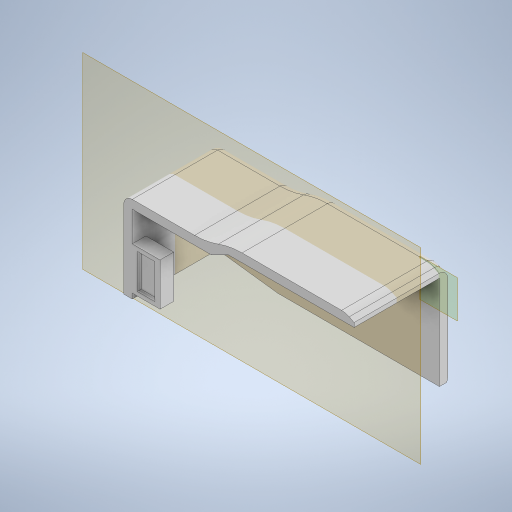
# Autodesk Inventor part: gondola
Saved by Autodesk Inventor 2023 (Build 270158000, 158)
## iProperties
Created: 2023-09-16
Part Number: gondola
Material: Generic
Document SubType Name: Modeling
Designer: alexa
Density: 1 g/cm^3
Appearance: Default
Author: alexa
Autodesk Inventor part; units mm, degrees
ref_plane "YZ Plane" through (0, 0, 0) normal (1, 0, 0) x (0, 1, 0)
ref_plane "XZ Plane" through (0, 0, 0) normal (0, 1, 0) x (-1, 0, 0)
ref_plane "XY Plane" through (0, 0, 0) normal (0, 0, 1) x (1, 0, 0)
sketch "Sketch1" plane through (0, 0, 0) normal (0, 1, 0) x (-1, 0, 0)
  line L0 (-70, 30) -> (70, 30)
  line L1 (70, 30) -> (70, -30)
  line L2 (70, -30) -> (-70, -30)
  line L3 (-70, -30) -> (-70, 30)
  line L4 (-70, 30) -> (70, -30) construction
  line L5 (70, 30) -> (-70, -30) construction
  point P0 (0, 0)
  dimension "d0" = 140
  dimension "d1" = 60
  constraints: 12 end point, 2 midpoint, 2 parallel, 1 horizontal, 1 perpendicular
  measures "d0" distance of L1.end L2.end
  measures "d1" distance between parallel lines of L0 L2
extrude "Extrusion1" add sketch "Sketch1" along normal blind 60
sketch "Sketch2" plane through (0, 60, 0) normal (0, 1, 0) x (1, 0, 0)
  point P0 (0, 0)
sketch "Sketch3" plane through (0, 60, 0) normal (0, 1, 0) x (1, 0, 0)
  line L0 (70, 30) -> (-70, 30) projected
  line L1 (-70, -30) -> (70, -30) projected
  line L2 (70, 30) -> (-20, 30)
  line L3 (-20, 30) -> (-20, -30)
  line L4 (-20, -30) -> (70, -30)
  line L5 (70, -30) -> (70, 30)
  point P0 (0, 0)
  point P1 (70, -30)
  point P2 (-20, 30)
  dimension "d4" = 90
  constraints: 8 end point, 2 parallel, 1 horizontal, 1 perpendicular, 1 point on line
  measures "d4" distance of L4.end L3.end
extrude "Extrusion2" add sketch "Sketch3" along normal blind 5
chamfer "Chamfer2" distance 5 distance2 40 1 edges at (-70, 0, 0) measured on face at (-70, 20, -10)
sketch "Sketch8" plane through (70, 0, 30) normal (1, 0, 0) x (0, 0, -1)
  circle A0 centre (30, 32.5) radius 13.25
  line L0 (0, 0) -> (60, 0) projected
  line L1 (60, 0) -> (60, 65) projected
  line L2 (0, 65) -> (60, 65) projected
  point P0 (30, 0)
  point P1 (60, 32.5)
  dimension "d26" = 26.5
  dimension "d27" = 32.5
  dimension "d28" = 30
  dimension "d88" = 32.5
  constraints: 1 centre point, 1 midpoint
  measures "d26" diameter of A0
  measures "d27" distance from line of L0 A0.centre
  measures "d28" distance of point (60, 32.5) A0.centre
  measures "d88" distance from line of L2 A0.centre
extrude "Extrusion6" cut sketch "Sketch8" against normal blind 10
sketch "Sketch9" plane through (70, 0, -30) normal (0, 0, -1) x (-1, 0, 0)
  line L0 (5, 60) -> (5, 5)
  line L1 (5, 5) -> (99.688711, 5)
  line L2 (99.688711, 5) -> (135, 9.413911)
  line L3 (135, 9.413911) -> (135, 55)
  line L4 (135, 55) -> (88.81966, 55)
  line L5 (88.81966, 55) -> (78.81966, 60)
  line L6 (78.81966, 60) -> (5, 60)
  line L7 (0, 65) -> (90, 65)
  line L8 (50, 80) -> (90, 60)
  line L9 (90, 60) -> (140, 60)
  line L10 (140, 5) -> (140, 60)
  line L11 (140, 5) -> (100, 0)
  line L12 (0, 0) -> (100, 0)
  line L13 (0, 0) -> (0, 65)
  point P0 (70, 0)
  dimension "d35" = 5
  dimension "d36" = 5
  dimension "d37" = 5
  dimension "d38" = 5
  dimension "d39" = 5
  dimension "d40" = 5
  dimension "d41" = 5
  constraints: 14 end point, 7 parallel, 2 perpendicular, 1 horizontal, 1 vertical, 1 other
  measures "d36" distance between parallel lines of L13 L0
  measures "d37" distance between parallel lines of L10 L3
  measures "d38" distance between parallel lines of L9 L4
  measures "d39" distance between parallel lines of L8 L5
  measures "d40" distance between parallel lines of L11 L2
  measures "d41" distance between parallel lines of L12 L1
extrude "Extrusion7" cut sketch "Sketch9" against normal blind 55 contours L6 L5 L4 L3 L2 L1 L0
ref_plane "Work Plane1" through (70, 0, 0) normal (0, 0, 1) x (1, 0, 0)
fillet "Fillet6" radius 5 1 edges at (-70, 60, 0)
fillet "Fillet9" radius 5 1 edges at (-70, 5, 0)
fillet "Fillet21" radius 40 1 edges at (-20, 65, 0)
fillet "Fillet22" radius 40 1 edges at (-20, 60, 0)
chamfer "Chamfer3" distance 10 distance2 5 1 edges at (70, 65, 0) measured on face at (46.455, 65, 10)
fillet "Fillet23" radius 5 1 edges at (70, 60, 0)
fillet "Fillet24" radius 10 1 edges at (60, 65, 0)
chamfer "Chamfer4" distance 5 distance2 10 1 edges at (70, 0, 0) measured on face at (70, 6.4489, -0.5324)
fillet "Fillet25" radius 10 1 edges at (60, 0, 0)
fillet "Fillet26" radius 5 1 edges at (70, 5, 0)
fillet "Fillet27" radius 5 15 edges at (59.9368, 64.7325, 30) (64.6738, 62.6631, 30) (69.2533, 59.5385, 30) (70, 32.5, 30) (69.2533, 5.4615, 30) (64.6738, 2.3369, 30) (59.9368, 0.2675, 30) (13.8197, 0, 30) (-7.7062, 64.37, 30) (-21.4028, 60.63, 30) (-46.737, 60, 30) (-70, 32.207, 30) (-68.7484, 6.1049, 30) (-47.8101, 2.2263, 30) (28.5021, 65, 30)
ref_plane "Work Plane7" through (65, 55, -24.5) normal (0, 0, -1) x (-1, 0, 0)
sketch "Sketch24" plane through (65, 55, -24.5) normal (0, 0, -1) x (-1, 0, 0)
  line L0 (0, 0) -> (5, 0) projected
  line L1 (5, 5) -> (5, 0) projected
  line L2 (5, 0) -> (5, 5) projected
  line L3 (0, 0) -> (0, 5) projected
  line L4 (5, 5) -> (0, 0)
  line L5 (5, -45) -> (5, -50) projected
  line L6 (0, -45) -> (5, -45) projected
  line L7 (0, -50) -> (0, -45) projected
  line L8 (0, -45) -> (5, -50)
  point P0 (65, -55)
  constraints: 4 end point
extrude "Extrusion21" cut sketch "Sketch24" against normal blind 5
sketch "Sketch27" plane through (65, 5, -30) normal (-1, 0, 0) x (0, 0, 1)
  line L0 (8.5, 30) -> (13.5, 30)
  line L1 (13.5, 30) -> (13.5, 25)
  line L2 (13.5, 25) -> (8.5, 25)
  line L3 (8.5, 25) -> (8.5, 30)
  line L4 (8.5, 30) -> (13.5, 25) construction
  line L5 (13.5, 30) -> (8.5, 25) construction
  circle A0 centre (30, 27.5) radius 13.25 projected
  line L6 (30, 73) -> (30, -18) projected
  line L7 (51.5, 30) -> (46.5, 30)
  line L8 (46.5, 30) -> (46.5, 25)
  line L9 (46.5, 25) -> (51.5, 25)
  line L10 (51.5, 25) -> (51.5, 30)
  point P0 (30, -5)
  point P1 (11, 27.5)
  dimension "d137" = 0
  dimension "d138" = 19
  dimension "d139" = 5
  dimension "d140" = 5
  constraints: 20 end point, 4 symmetric about line, 2 midpoint, 2 parallel, 1 horizontal, 1 perpendicular
  measures "d137" vertical distance of A0.centre point (11, 27.5)
  measures "d138" distance of A0.centre point (11, 27.5)
  measures "d139" distance of L2.end L0.start
  measures "d140" distance of L0.start L0.end
extrude "Extrusion24" add sketch "Sketch27" along normal blind 10 contours L0 L1 L2 L3 | L10 L9 L8 L7
sketch "Sketch28" plane through (65, 30, 16.5) normal (0, 0, -1) x (-1, 0, 0)
  line L0 (0, 5) -> (10, 5) projected
  line L1 (0, 0) -> (10, 0) projected
  line L2 (10, 5) -> (5, 5)
  line L3 (5, 5) -> (5, 0)
  line L4 (5, 0) -> (10, 0)
  line L5 (10, 0) -> (10, 5)
  point P0 (65, -30)
  point P1 (5, 5)
  dimension "d143" = 5
  constraints: 8 end point, 2 parallel, 1 horizontal, 1 midpoint, 1 perpendicular
  measures "d143" distance between parallel lines of L5 L3
extrude "Extrusion25" add sketch "Sketch28" along normal up to surface (33 mm away)
sketch "Sketch29" plane through (55, 5, -30) normal (-1, 0, 0) x (0, 0, 1)
  line L0 (30, 73) -> (30, -18) projected
  circle A0 centre (25.5, 27.5) radius 1.5
  line L1 (51.5, 30) -> (8.5, 30) projected
  line L2 (8.5, 25) -> (51.5, 25) projected
  circle A1 centre (34.5, 27.5) radius 1.5
  point P0 (30, -5)
  dimension "d146" = 4.5
  dimension "d147" = 3
  dimension "d148" = 2.5
  dimension "d149" = 2.5
  constraints: 2 centre point, 1 symmetric about line, 1 other
  measures "d146" distance from line of A0.centre L0
  measures "d147" diameter of A0
  measures "d148" distance from line of L1 A0.centre
  measures "d149" distance from line of L2 A0.centre
extrude "Extrusion26" cut sketch "Sketch29" against normal up to surface (5 mm away)
sketch "Sketch30" plane through (55, 5, -30) normal (-1, 0, 0) x (0, 0, 1)
  line L0 (30, 73) -> (30, -18) projected
  circle A0 centre (30, 27.5) radius 3.5
  line L1 (51.5, 30) -> (8.5, 30) projected
  point P0 (30, -5)
  dimension "d152" = 2.5
  dimension "d153" = 7
  constraints: 1 centre point, 1 midpoint
  measures "d152" distance from line of L1 A0.centre
  measures "d153" diameter of A0
extrude "Extrusion27" cut sketch "Sketch30" against normal up to surface (5 mm away)
sketch "Sketch32" plane through (0, 0, 0) normal (0, -1, 0) x (1, 0, 0)
  circle A0 centre (20, 0) radius 14.25
  line L0 (65, -30) -> (65, 25) projected
  point P0 (0, 0)
  point P1 (65, -21.5)
  dimension "d158" = 28.5
  dimension "d159" = 45
  constraints: 1 centre point
  measures "d158" diameter of A0
  measures "d159" distance from line of A0.centre L0
extrude "Extrusion29" cut sketch "Sketch32" against normal blind 5
ref_plane "Work Plane4" through (0, 32.5, 0) normal (0, -1, 0) x (1, 0, 0)
sketch "Sketch34" plane through (-29.688711, 5, -30) normal (0, 1, 0) x (1, 0, 0)
  line L0 (15.188711, -15.5) -> (8.188711, -15.5)
  line L1 (8.188711, -15.5) -> (8.188711, -8.5)
  line L2 (8.188711, -8.5) -> (15.188711, -8.5)
  line L3 (15.188711, -8.5) -> (15.188711, -15.5)
  line L4 (15.188711, -15.5) -> (8.188711, -8.5) construction
  line L5 (8.188711, -15.5) -> (15.188711, -8.5) construction
  line L6 (127.688711, -30) -> (-68.311289, -30)
  circle A0 centre (49.688711, -30) radius 14.25
  line L7 (15.188711, -44.5) -> (8.188711, -44.5)
  line L8 (8.188711, -44.5) -> (8.188711, -51.5)
  line L9 (8.188711, -51.5) -> (15.188711, -51.5)
  line L10 (15.188711, -51.5) -> (15.188711, -44.5)
  point P0 (29.688711, -30)
  point P1 (11.688711, -12)
  dimension "d163" = 7
  dimension "d164" = 7
  dimension "d166" = 18
  dimension "d167" = 38
  constraints: 20 end point, 4 symmetric about line, 2 midpoint, 2 parallel, 1 horizontal, 1 perpendicular
  measures "d163" distance between parallel lines of L2 L0
  measures "d164" distance between parallel lines of L1 L3
  measures "d166" distance from line of L6 point (11.689, -12)
  measures "d167" horizontal distance of A0.centre point (11.689, -12)
extrude "Extrusion30" add sketch "Sketch34" along normal blind 12 contours L0 L1 L2 L3 | L10 L9 L8 L7
sketch "Sketch35" plane through (-29.688711, 17, -30) normal (0, 1, 0) x (1, 0, 0)
  circle A0 centre (11.688711, -48) radius 2
  line L0 (8.188711, -44.5) -> (8.188711, -51.5)
  line L1 (15.188711, -44.5) -> (8.188711, -44.5)
  line L2 (15.188711, -51.5) -> (15.188711, -44.5)
  line L3 (127.688711, -30) -> (-68.311289, -30)
  circle A1 centre (11.688711, -12) radius 2
  point P0 (29.688711, -30)
  dimension "d170" = 4
  dimension "d171" = 3.5
  dimension "d172" = 3.5
  dimension "d173" = 3.5
  constraints: 2 centre point, 1 symmetric about line, 1 other
  measures "d170" diameter of A0
  measures "d171" distance from line of A0.centre L0
  measures "d172" distance from line of L1 A0.centre
  measures "d173" distance from line of L2 A0.centre
extrude "Extrusion31" cut sketch "Sketch35" against normal blind 5
sketch "Sketch37" plane through (-29.688711, 5, -30) normal (0, 1, 0) x (1, 0, 0)
  line L0 (8.188711, -51.5) -> (8.188711, -44.5)
  line L1 (0, -55) -> (94.688711, -55)
  line L2 (8.188711, -51.5) -> (15.188711, -51.5)
  line L3 (15.188711, -51.5) -> (15.188711, -55)
  line L4 (15.188711, -55) -> (8.188711, -55)
  line L5 (8.188711, -55) -> (8.188711, -51.5)
  line L6 (15.188711, -44.5) -> (15.188711, -51.5)
  point P0 (29.688711, -30)
  point P1 (8.188711, -55)
  dimension "d178" = 0
  constraints: 8 end point, 2 parallel, 1 collinear, 1 horizontal, 1 perpendicular, 1 point on line
  measures "d178" distance between parallel lines of L6 L3
extrude "Extrusion32" add sketch "Sketch37" along normal blind 12
sketch "Sketch38" plane through (65, 30, 21.5) normal (0, 0, 1) x (1, 0, 0)
  line L0 (0, 5) -> (0, 0) projected
  line L1 (0, 5) -> (-10, 5) projected
  line L2 (-10, 0) -> (-10, 5) projected
  line L3 (0, 0) -> (-10, 0) projected
  point P0 (-65, -30)
extrude "Extrusion33" add sketch "Sketch38" along normal up to surface (3.5 mm away)
ref_plane "Work Plane6" through (-70, 9.413911, -22.5) normal (0, 0, -1) x (-1, 0, 0)
ref_plane "Work Plane5" through (-70, 9.413911, -15) normal (0, 0, -1) x (-1, 0, 0)
sketch "Sketch42" plane through (55, 5, -30) normal (-1, 0, 0) x (0, 0, 1)
  line L0 (22.5, 34) -> (37.5, 34)
  line L1 (37.5, 34) -> (37.5, 21)
  line L2 (37.5, 21) -> (22.5, 21)
  line L3 (22.5, 21) -> (22.5, 34)
  arc A0 (32.44949, 25) -> (33.361111, 26.523818) centre (30, 27.5) ccw
  line L4 (22.5, 34) -> (37.5, 21) construction
  line L5 (37.5, 34) -> (22.5, 21) construction
  point P0 (30, -5)
  dimension "d193" = 15
  dimension "d194" = 13
  constraints: 12 end point, 2 midpoint, 2 parallel, 1 horizontal, 1 perpendicular
  measures "d193" distance of L0.start L0.end
  measures "d194" distance of L0.end L1.end
extrude "Extrusion36" add sketch "Sketch42" against normal blind 5
sketch "Sketch43" plane through (55, 5, -30) normal (-1, 0, 0) x (0, 0, 1)
  line L0 (24, 32.5) -> (36, 32.5)
  line L1 (36, 32.5) -> (36, 22.5)
  line L2 (36, 22.5) -> (24, 22.5)
  line L3 (24, 22.5) -> (24, 32.5)
  circle A0 centre (30, 27.5) radius 2.15 projected
  line L4 (24, 32.5) -> (36, 22.5) construction
  line L5 (36, 32.5) -> (24, 22.5) construction
  point P0 (30, -5)
  dimension "d197" = 12
  dimension "d199" = 10
  constraints: 12 end point, 2 midpoint, 2 parallel, 1 horizontal, 1 perpendicular
  measures "d197" distance of L0.start L0.end
  measures "d199" distance of L0.end L1.end
extrude "Extrusion37" cut sketch "Sketch43" against normal blind 2.5
sketch "Sketch44" plane through (55, 5, -30) normal (-1, 0, 0) x (0, 0, 1)
  line L0 (22.5, 25) -> (22.5, 21) projected
  line L1 (8.5, 25) -> (22.5, 25) projected
  line L2 (22.5, 21) -> (18.5, 25)
  point P0 (30, -5)
  dimension "d202" = 45
  dimension "d203" = 45
  constraints: 2 end point, 1 point on line
  measures "d202" angle of L1 L2
  measures "d203" angle of L0 L2
extrude "Extrusion38" add sketch "Sketch44" against normal blind 5
mirror "Mirror1" about plane through (70, 0, 0) normal (0, 0, 1) of "Extrusion38"
sketch "Sketch45" plane through (55, 5, -30) normal (-1, 0, 0) x (0, 0, 1)
  line L0 (37.5, 34) -> (22.5, 34) projected
  line L1 (22.5, 34) -> (18.5, 30)
  line L2 (8.5, 30) -> (22.5, 30) projected
  line L3 (22.5, 34) -> (22.5, 30) projected
  point P0 (30, -5)
  dimension "d206" = 45
  dimension "d207" = 45
  constraints: 2 end point, 1 point on line
  measures "d206" angle of L2 L1
  measures "d207" angle of L1 L3
extrude "Extrusion39" add sketch "Sketch45" against normal blind 5
mirror "Mirror2" about plane through (70, 0, 0) normal (0, 0, 1) of "Extrusion39"
sketch "Sketch46" plane through (55, 32.5, 0) normal (-1, 0, 0) x (0, 0, 1)
  circle A0 centre (0, 0) radius 4
  point P0 (0, -32.5)
  dimension "d210" = 8
  constraints: 1 centre point
  measures "d210" diameter of A0
extrude "Extrusion40" cut sketch "Sketch46" against normal blind 5
sketch "Sketch47" plane through (70, 0, 25) normal (0, 0, -1) x (-1, 0, 0)
  line L0 (5, 35) -> (15, 35)
  line L1 (15, 35) -> (15, 30)
  line L2 (15, 30) -> (5, 30)
  line L3 (5, 5) -> (5, 30)
  line L4 (84.5, 5) -> (5, 5)
  line L5 (84.5, 5) -> (84.5, 17)
  line L6 (84.5, 17) -> (91.5, 17)
  line L7 (91.5, 17) -> (91.5, 5)
  line L8 (99.688711, 5) -> (91.5, 5)
  line L9 (135, 9.413911) -> (99.688711, 5)
  line L10 (135, 55) -> (135, 9.413911)
  line L11 (88.81966, 55) -> (135, 55)
  line L12 (78.81966, 60) -> (88.81966, 55)
  line L13 (5, 60) -> (78.81966, 60)
  line L14 (5, 35) -> (5, 60)
  line L15 (91.5, 5) -> (84.5, 5)
  point P0 (70, 0)
extrude "Extrusion41" cut sketch "Sketch47" against normal blind 10
sketch "Sketch48" plane through (-70, 9.413911, -30) normal (0, 0, -1) x (-1, 0, 0)
  line L0 (-135, 50.586089) -> (-61.18034, 50.586089)
  line L1 (-61.18034, 50.586089) -> (-51.18034, 45.586089)
  line L2 (-51.18034, 45.586089) -> (-5, 45.586089)
  line L3 (-5, 45.586089) -> (-5, 0)
  line L4 (-5, 0) -> (-40.311289, -4.413911)
  line L5 (-40.311289, -4.413911) -> (-135, -4.413911)
  line L6 (-135, -4.413911) -> (-135, 50.586089)
  point P0 (-70, -9.413911)
extrude "Extrusion42" add sketch "Sketch48" against normal blind 5
fillet "Fillet29" radius 5 16 edges at (-7.7062, 64.37, -30) (-21.4028, 60.63, -30) (-46.737, 60, -30) (-68.5355, 58.5355, -30) (-70, 32.207, -30) (-68.7484, 6.1049, -30) (-47.8101, 2.2263, -30) (59.9368, 64.7325, -30) (64.6738, 62.6631, -30) (69.2533, 59.5385, -30) (70, 32.5, -30) (69.2533, 5.4615, -30) (64.6738, 2.3369, -30) (59.9368, 0.2675, -30) (13.8197, 0, -30) (28.5021, 65, -30)
sketch "Sketch50" plane through (70, 8.09017, 25) normal (1, 0, 0) x (0, 0, -1)
  line L0 (50, -3.09017) -> (-4.166615, -3.09017)
  line L1 (-5, 21.90983) -> (-5, 0)
  line L2 (-5, 48.81966) -> (-5, 26.90983)
  line L3 (-5, 26.90983) -> (-5, 21.90983)
  ellipse E0 centre (0, 0) end of major axis (0, -5.59017) minor radius 5 (-5, 0) -> (-4.166615, -3.09017) ccw
  line L4 (50, 51.90983) -> (-4.166615, 51.90983)
  line L5 (55, 0) -> (55, 48.81966)
  ellipse E1 centre (50, 0) end of major axis (55, 0) minor radius 4.472136 (50, -4.472136) -> (55, 0) ccw
  line L6 (46.5, 51.90983) -> (55, 51.90983)
  line L7 (55, 51.90983) -> (55, 48.23178)
  line L8 (-4.166615, 51.90983) -> (-5, 51.90983)
  ellipse E2 centre (0, 48.81966) end of major axis (-5, 48.81966) minor radius 4.472136 (0, 53.291796) -> (-5, 48.81966) ccw
  line L9 (-5, 51.90983) -> (-5, 48.81966)
  line L10 (46.5, -3.09017) -> (53.614355, -3.09017)
  line L11 (50, 48.81966) -> (50, 0)
  line L12 (50, -4.472136) -> (50, 0)
  line L13 (50, 48.81966) -> (50, 53.291796)
  point P0 (25, -8.09017)
  point P1 (-3.614355, 51.90983)
  constraints: 10 end point, 2 horizontal, 2 point on line, 2 vertical, 4 other
sketch "Sketch51" plane through (-0.635083, 60, 30) normal (0, -1, 0) x (1, 0, 0)
  line L0 (65.635083, -55) -> (65.635083, -0.833385)
  line L1 (70.635083, -5) -> (70.635083, -55)
  line L2 (70.635083, -51.5) -> (70.635083, -0.833385)
  line L3 (65.635083, -0.833385) -> (70.635083, -0.833385)
  line L4 (58.274403, 0) -> (-29.053628, 0)
  line L5 (-8.184577, -55) -> (65.635083, -55)
  line L6 (70.635083, -60) -> (65.635083, -55)
  line L7 (70.635083, -60) -> (65.635083, -55)
  line L8 (67.871151, -55) -> (70.635083, -55)
  line L9 (65.635083, -55) -> (70.635083, -55)
  point P0 (0.635083, -30)
  point P1 (65.635083, -51.5)
  point P2 (65.635083, -55)
  point P3 (67.871151, -55)
  constraints: 8 end point, 1 collinear, 1 parallel
extrude "Extrusion43" cut sketch "Sketch50" against normal blind 50 contours L0 E0 L1 L3 L2 E2 L4 L13 L11 L12
extrude "Extrusion44" cut sketch "Sketch51" against normal blind 50
sketch "Sketch52" plane through (-0.635083, 60, 30) normal (0, 1, 0) x (1, 0, 0)
  line L0 (67.180168, 1.385645) -> (65.635083, 1.385645)
  line L1 (65.635083, 1.385645) -> (68.166593, 1.385645)
  line L2 (68.166593, 1.385645) -> (68.166593, -1.6054)
  line L3 (68.166593, -1.6054) -> (65.635083, -1.6054)
  line L4 (65.635083, -1.6054) -> (65.635083, 1.385645)
  point P0 (0.635083, 30)
  point P1 (67.180168, 1.385645)
  constraints: 8 end point, 2 parallel, 1 horizontal, 1 perpendicular
extrude "Extrusion45" cut sketch "Sketch52" against normal blind 10
sketch "Sketch53" plane through (-70, 9.413911, 25) normal (-1, 0, 0) x (0, 0, 1)
  line L0 (-50, 0) -> (-50, 45.586089)
  line L1 (-50, 0) -> (13.21215, 0)
  line L2 (13.21215, 0) -> (13.21215, -27.239503)
  line L3 (13.21215, -27.239503) -> (-50, -27.239503)
  line L4 (-50, -27.239503) -> (-50, 0)
  point P0 (-25, -9.413911)
  constraints: 8 end point, 2 parallel, 1 horizontal, 1 perpendicular
extrude "Extrusion46" cut sketch "Sketch53" against normal blind 200
sketch "Sketch54" plane through (-14.5, 17, 25) normal (1, 0, 0) x (0, 0, -1)
  line L0 (0, 0) -> (10.5, 0)
  line L1 (0, 0) -> (47.590826, 0)
  line L2 (47.590826, 0) -> (47.590826, -20.025121)
  line L3 (47.590826, -20.025121) -> (0, -20.025121)
  line L4 (0, -20.025121) -> (0, 0)
  point P0 (25, -17)
  point P1 (10.5, 0)
  constraints: 8 end point, 2 parallel, 1 horizontal, 1 perpendicular
extrude "Extrusion47" cut sketch "Sketch54" against normal blind 10
sketch "Sketch55" plane through (57.63932, 5, -30) normal (0, 0, -1) x (-1, 0, 0)
  line L0 (122.63932, 4.413911) -> (87.328031, 0)
  line L1 (127.63932, 4.413911) -> (122.63932, 4.413911)
  line L2 (87.328031, 0) -> (0, 0)
  line L3 (-7.36068, 55) -> (-7.36068, 57.5)
  line L4 (-7.36068, 3.09017) -> (-7.36068, 51.90983)
  line L5 (-7.36068, 51.90983) -> (-7.36068, 55)
  line L6 (-9.596748, -1.381966) -> (-7.36068, 3.09017)
  line L7 (-7.36068, 3.09017) -> (-7.36068, 0)
  arc A0 (-2.236068, 0.527864) -> (0, 0) centre (0, 5) ccw
  line L8 (-7.36068, 0) -> (0, 0)
  arc A1 (-9.596748, 56.381966) -> (-12.36068, 51.90983) centre (-7.36068, 51.90983) ccw
  line L9 (-12.36068, 51.90983) -> (-12.36068, 3.09017)
  arc A2 (-12.36068, 3.09017) -> (-9.596748, -1.381966) centre (-7.36068, 3.09017) ccw
  line L10 (-9.596748, -1.381966) -> (-4.472136, -3.944272)
  arc A3 (-4.472136, -3.944272) -> (0, -5) centre (0, 5) ccw
  line L11 (0, -5) -> (87.63932, -5)
  line L12 (87.63932, -5) -> (123.259494, -0.547478)
  arc A4 (123.259494, -0.547478) -> (127.63932, 4.413911) centre (122.63932, 4.413911) ccw
  line L13 (-7.36068, 57.5) -> (-9.596748, 56.381966)
  point P0 (57.63932, -5)
  constraints: 6 end point, 1 perpendicular, 1 point on line, 1 tangent, 1 vertical
extrude "Extrusion48" cut sketch "Sketch55" against normal blind 10
sketch "Sketch56" plane through (65, 60, 29.166615) normal (1, 0, 0) x (0, 0, -1)
  arc A0 (4.166615, 5) -> (-0.833385, 0) centre (4.166615, 0) ccw
  line L0 (4.166615, 5) -> (-2.994967, 5)
  line L1 (-2.994967, 5) -> (-2.994967, -58.255247)
  line L2 (-2.994967, -58.255247) -> (4.166615, -58.255247)
  line L3 (4.166615, -58.255247) -> (4.166615, 5)
  point P0 (29.166615, -60)
  constraints: 8 end point, 2 parallel, 1 horizontal, 1 perpendicular
extrude "Extrusion49" cut sketch "Sketch56" against normal through all
sketch "Sketch57" plane through (-8.81966, 60, -25) normal (0, -1, 0) x (1, 0, 0)
  line L0 (28.81966, 34.5) -> (48.81966, 34.5)
  line L1 (48.81966, 34.5) -> (48.81966, 45)
  line L2 (48.81966, 45) -> (28.81966, 45)
  line L3 (28.81966, 45) -> (28.81966, 34.5)
  line L4 (73.81966, 0) -> (73.81966, 50)
  line L5 (73.81966, 50) -> (0, 50)
  point P0 (8.81966, 25)
  point P1 (48.81966, 39.75)
  point P2 (36.90983, 50)
  dimension "d232" = 25
  dimension "d233" = 15.5
  dimension "d234" = 5
  dimension "d235" = 20
  constraints: 8 end point, 2 midpoint, 2 parallel, 1 horizontal, 1 perpendicular
  measures "d232" distance from line of L4 point (48.82, 39.75)
  measures "d233" distance from line of point (36.91, 50) L0
  measures "d234" distance between parallel lines of L5 L2
  measures "d235" distance between parallel lines of L1 L3
extrude "Extrusion50" cut sketch "Sketch57" against normal blind 2.7
sketch "Sketch58" plane through (-65, 9.413911, -25) normal (1, 0, 0) x (0, 0, -1)
  line L0 (-50, 28) -> (-42, 28)
  line L1 (-42, 28) -> (-42, 3)
  line L2 (-42, 3) -> (-50, 3)
  line L3 (-50, 3) -> (-50, 28)
  line L4 (0, 0) -> (-50, 0)
  line L5 (-50, 45.586089) -> (-50, 0)
  point P0 (-25, -9.413911)
  dimension "d238" = 8
  dimension "d239" = 3
  dimension "d240" = 0
  dimension "d241" = 25
  constraints: 8 end point, 2 parallel, 1 horizontal, 1 perpendicular
  measures "d238" distance between parallel lines of L1 L3
  measures "d239" distance between parallel lines of L4 L2
  measures "d240" distance between parallel lines of L5 L3
  measures "d241" distance between parallel lines of L2 L0
extrude "Extrusion51" add sketch "Sketch58" along normal blind 22
sketch "Sketch59" plane through (-8.81966, 60, 25) normal (0, 0, 1) x (1, 0, 0)
  line L0 (-53.18034, -24.936089) -> (-42.88034, -24.936089)
  line L1 (-42.88034, -24.936089) -> (-42.88034, -45.236089)
  line L2 (-42.88034, -45.236089) -> (-53.18034, -45.236089)
  line L3 (-53.18034, -45.236089) -> (-53.18034, -24.936089)
  line L4 (-56.18034, -5) -> (-56.18034, -22.586089)
  line L5 (-61.18034, -5) -> (-61.18034, -50.586089)
  line L6 (-56.18034, -47.586089) -> (-34.18034, -47.586089)
  line L7 (-56.18034, -22.586089) -> (-34.18034, -22.586089)
  point P0 (8.81966, -60)
  dimension "d245" = 8
  dimension "d246" = 10.3
  dimension "d247" = 20.3
  dimension "d248" = 2.35
  dimension "d249" = 2.35
  constraints: 8 end point, 2 parallel, 1 horizontal, 1 perpendicular
  measures "d245" distance between parallel lines of L5 L3
  measures "d246" distance between parallel lines of L3 L1
  measures "d247" distance between parallel lines of L2 L0
  measures "d248" distance between parallel lines of L6 L2
  measures "d249" distance between parallel lines of L7 L0
extrude "Extrusion52" cut sketch "Sketch59" against normal blind 2.2
sketch "Sketch60" plane through (-43, 9.413911, -25) normal (1, 0, 0) x (0, 0, -1)
  line L0 (-42, 28) -> (-50, 28) projected
  line L1 (-50, 28) -> (-50, 3) projected
  line L2 (-50, 3) -> (-42, 3) projected
  line L3 (-42, 3) -> (-42, 28) projected
  point P0 (-25, -9.413911)
extrude "Extrusion53" cut sketch "Sketch60" against normal blind 5.7
body "Solid1"
